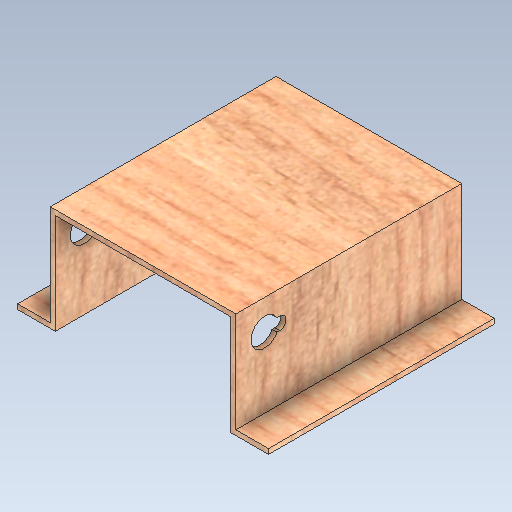
# Autodesk Inventor part: wc
Saved by Autodesk Inventor 2021 (Build 250183000, 183)
## iProperties
Created: 2021-07-06
Part Number: wc
Material: Wood (Birch)
Document SubType Name: Modeling
Designer: KAVYA
Density: 0.55 g/cm^3
Appearance: Birch - Natural Polished
Author: KAVYA
Autodesk Inventor part; units mm, degrees
ref_plane "YZ Plane" through (0, 0, 0) normal (1, 0, 0) x (0, 1, 0)
ref_plane "XZ Plane" through (0, 0, 0) normal (0, 1, 0) x (-1, 0, 0)
ref_plane "XY Plane" through (0, 0, 0) normal (0, 0, 1) x (1, 0, 0)
sketch "Sketch1" plane through (0, 0, 0) normal (0, 1, 0) x (-1, 0, 0)
  line L0 (0, 0) -> (-70, 0)
  line L1 (-70, 0) -> (-70, -90)
  line L2 (-70, -90) -> (0, -90)
  line L3 (0, -90) -> (0, 0)
  dimension "d0" = 70
  dimension "d1" = 90
  constraints: 8 end point, 2 parallel, 1 horizontal, 1 perpendicular
  measures "d0" distance of L2.end L1.end
  measures "d1" distance of L1.end L0.end
extrude "Extrusion1" add sketch "Sketch1" along normal blind 2
sketch "Sketch2" plane through (70, 0, 0) normal (1, 0, 0) x (0, 0, -1)
  line L0 (0, 2) -> (90, 2) projected
  line L1 (0, 2) -> (90, 2)
  line L2 (90, 2) -> (90, -38)
  line L3 (90, -38) -> (0, -38)
  line L4 (0, -38) -> (0, 2)
  point P0 (0, 0)
  dimension "d4" = 90
  dimension "d5" = 40
  constraints: 8 end point, 2 parallel, 1 horizontal, 1 perpendicular
  measures "d4" distance of L2.end L3.end
  measures "d5" distance of L1.end L2.end
extrude "Extrusion2" add sketch "Sketch2" along normal blind 2
sketch "Sketch3" plane through (0, 0, -90) normal (-1, 0, 0) x (0, 0, 1)
  line L0 (0, 2) -> (90, 2) projected
  line L1 (90, -38) -> (0, -38) projected
  line L2 (0, 2) -> (90, 2)
  line L3 (90, 2) -> (90, -38)
  line L4 (90, -38) -> (0, -38)
  line L5 (0, -38) -> (0, 2)
  point P0 (90, 0)
  constraints: 8 end point, 2 parallel, 1 horizontal, 1 perpendicular
extrude "Extrusion3" add sketch "Sketch3" along normal blind 2
sketch "Sketch4" plane through (70, -38, -90) normal (0, -1, 0) x (1, 0, 0)
  line L0 (0, 90) -> (0, 0) projected
  line L1 (0, 0) -> (15, 0)
  line L2 (15, 0) -> (15, 90)
  line L3 (15, 90) -> (0, 90)
  line L4 (0, 90) -> (0, 0)
  line L5 (-70, 0) -> (-70, 90) projected
  line L6 (-70, 0) -> (-85, 0)
  line L7 (-85, 0) -> (-85, 90)
  line L8 (-85, 90) -> (-70, 90)
  line L9 (-70, 90) -> (-70, 0)
  dimension "d10" = 15
  dimension "d11" = 15
  constraints: 16 end point, 4 parallel, 2 horizontal, 2 perpendicular
  measures "d10" distance of L3.end L2.end
  measures "d11" distance of L7.end L8.end
extrude "Extrusion4" add sketch "Sketch4" along normal blind 2
sketch "Sketch5" plane through (72, 0, 0) normal (1, 0, 0) x (0, 0, -1)
  arc A0 (16.399, -7.5) -> (16.399, -12.5) centre (11.5, -10) ccw
  line L0 (0, 2) -> (0, -38) projected
  line L1 (0, 0) -> (90, 0) projected
  arc A1 (17.5, -12.5) -> (17.5, -7.5) centre (17.5, -10) ccw
  line L2 (17.5, -7.5) -> (16.399, -7.5)
  line L3 (17.5, -12.5) -> (16.399, -12.5)
  dimension "d14" = 11
  dimension "d15" = 11.5
  dimension "d18" = 5
  constraints: 4 end point, 4 point on circle, 2 centre point, 2 tangent
  measures "d14" diameter of A0
  measures "d15" distance from line of L0 A0.centre
  measures "d18" diameter of A1
extrude "Extrusion5" cut sketch "Sketch5" against normal blind 95
body "Solid1"
